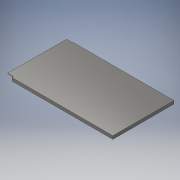
# Autodesk Inventor part: Display Controller
Saved by Autodesk Inventor 2017 SP1 (Build 210196100, 196)
## iProperties
Part Number: Display Controller
Material: Stahl, galvanisiert
Document SubType Name: Modeling
Designer: u26048
Density: 7.85 g/cm^3
Appearance: Galvanisiert
Author: u26048
Autodesk Inventor part; units mm, degrees
ref_plane "YZ Plane" through (0, 0, 0) normal (1, 0, 0) x (0, 1, 0)
ref_plane "XZ Plane" through (0, 0, 0) normal (0, 1, 0) x (-1, 0, 0)
ref_plane "XY Plane" through (0, 0, 0) normal (0, 0, 1) x (1, 0, 0)
sketch "Skizze1" plane through (0, 0, 0) normal (0, 0, 1) x (1, 0, 0)
  line L0 (-83.1, 50.3) -> (83.1, 50.3)
  line L1 (83.1, 50.3) -> (83.1, -50.3)
  line L2 (83.1, -50.3) -> (-83.1, -50.3)
  line L3 (-83.1, -50.3) -> (-83.1, 50.3)
  point P0 (0, 0)
  point P1 (83.1, 0)
  point P2 (0, 50.3)
  dimension "d0" = 166.2
  dimension "d1" = 100.6
  constraints: 8 end point, 2 midpoint, 2 parallel, 1 horizontal, 1 horizontal alignment, 1 perpendicular, 1 vertical alignment
  measures "d0" distance of L1.end L2.end
  measures "d1" distance of L0.end L1.end
extrude "Extrusion1" add sketch "Skizze1" along normal blind 5.26
sketch "Skizze2" plane through (0, 0, 0) normal (0, 0, -1) x (-1, 0, 0)
  line L0 (-83.1, 50.3) -> (-83.1, -50.3) projected
  line L1 (83.1, -50.3) -> (83.1, 50.3) projected
  line L2 (83.1, 50.3) -> (-83.1, 50.3) projected
  line L3 (-70.6, 31.6) -> (-55.6, 31.6)
  line L4 (-55.6, 31.6) -> (-55.6, 39.1)
  line L5 (-55.6, 39.1) -> (-70.6, 39.1)
  line L6 (-70.6, 39.1) -> (-70.6, 31.6)
  line L7 (-70.6, 31.6) -> (-55.6, 39.1) construction
  line L8 (-55.6, 31.6) -> (-70.6, 39.1) construction
  circle A0 centre (-63.1, 35.35) radius 1.5
  line L9 (55.6, 31.6) -> (70.6, 31.6)
  line L10 (70.6, 31.6) -> (70.6, 39.1)
  line L11 (70.6, 39.1) -> (55.6, 39.1)
  line L12 (55.6, 39.1) -> (55.6, 31.6)
  line L13 (55.6, 31.6) -> (70.6, 39.1) construction
  line L14 (70.6, 31.6) -> (55.6, 39.1) construction
  circle A1 centre (63.1, 35.35) radius 1.5
  line L15 (-55.6, -34.05) -> (-55.6, -26.55)
  circle A2 centre (-63.1, -30.3) radius 1.5
  line L16 (-70.6, -34.05) -> (-55.6, -34.05)
  line L17 (-70.6, -34.05) -> (-55.6, -26.55) construction
  line L18 (-55.6, -34.05) -> (-70.6, -26.55) construction
  line L19 (-55.6, -26.55) -> (-70.6, -26.55)
  line L20 (-70.6, -26.55) -> (-70.6, -34.05)
  line L21 (55.6, -26.55) -> (55.6, -34.05)
  circle A3 centre (63.1, -30.3) radius 1.5
  line L22 (70.6, -34.05) -> (70.6, -26.55)
  line L23 (70.6, -26.55) -> (55.6, -26.55)
  line L24 (55.6, -34.05) -> (70.6, -26.55) construction
  line L25 (70.6, -34.05) -> (55.6, -26.55) construction
  line L26 (55.6, -34.05) -> (70.6, -34.05)
  point P0 (0, 0)
  point P1 (63.1, 35.35)
  point P2 (-63.1, -30.3)
  point P3 (63.1, -30.3)
  point P4 (63.1, -30.3)
  dimension "d4" = 20
  dimension "d7" = 126.2
  dimension "d9" = 14.95
  dimension "d10" = 65.65
  dimension "d11" = 15
  dimension "d12" = 7.5
  dimension "d19" = 3
  dimension "d50" = 126.2
  dimension "d57" = 65.65
  constraints: 48 end point, 8 midpoint, 4 centre point, 4 coincident, 2 horizontal, 2 horizontal alignment, 2 parallel, 2 vertical alignment, 1 perpendicular, 1 vertical, 40 other
  measures "d4" distance from line of point (-63.1, 35.35) L0
  measures "d7" distance of point (63.1, 35.35) point (-63.1, 35.35)
  measures "d9" distance from line of L2 point (63.1, 35.35)
  measures "d10" distance of point (63.1, 35.35) point (63.1, -30.3)
  measures "d11" distance of L5.end L4.end
  measures "d12" distance of L4.end L3.end
  measures "d19" diameter of A0
  measures "d50" distance of L3.start L9.start
  measures "d57" distance of L3.end L15.start
extrude "Extrusion2" add sketch "Skizze2" along normal blind 2.5
sketch "Skizze3" plane through (0, 0, 0) normal (0, 0, -1) x (-1, 0, 0)
  line L0 (-82.45, 50.3) -> (82.45, 50.3)
  line L1 (82.45, 50.3) -> (82.45, -50.3)
  line L2 (82.45, -50.3) -> (-82.45, -50.3)
  line L3 (-82.45, -50.3) -> (-82.45, 50.3)
  line L4 (-37.75, 22) -> (-30.25, 22)
  line L5 (-30.25, 22) -> (-30.25, 37)
  line L6 (-30.25, 37) -> (-37.75, 37)
  line L7 (-37.75, 37) -> (-37.75, 22)
  line L8 (-37.75, 22) -> (-30.25, 37) construction
  line L9 (-30.25, 22) -> (-37.75, 37) construction
  circle A0 centre (-34, 29.5) radius 1.25
  line L10 (20.25, 22) -> (27.75, 22)
  line L11 (27.75, 22) -> (27.75, 37)
  line L12 (27.75, 37) -> (20.25, 37)
  line L13 (20.25, 37) -> (20.25, 22)
  line L14 (20.25, 22) -> (27.75, 37) construction
  line L15 (27.75, 22) -> (20.25, 37) construction
  circle A1 centre (24, 29.5) radius 1.25
  line L16 (-37.75, -27) -> (-30.25, -27)
  line L17 (-30.25, -27) -> (-30.25, -12)
  line L18 (-30.25, -12) -> (-37.75, -12)
  line L19 (-37.75, -12) -> (-37.75, -27)
  line L20 (-37.75, -27) -> (-30.25, -12) construction
  line L21 (-30.25, -27) -> (-37.75, -12) construction
  circle A2 centre (-34, -19.5) radius 1.25
  line L22 (20.25, -27) -> (27.75, -27)
  line L23 (27.75, -27) -> (27.75, -12)
  line L24 (27.75, -12) -> (20.25, -12)
  line L25 (20.25, -12) -> (20.25, -27)
  line L26 (20.25, -27) -> (27.75, -12) construction
  line L27 (27.75, -27) -> (20.25, -12) construction
  circle A3 centre (24, -19.5) radius 1.25
  point P0 (0, 0)
  point P1 (-82.45, 0)
  point P2 (0, 50.3)
  point P3 (-34, -19.5)
  point P4 (24, -19.5)
  dimension "d25" = 164.9
  dimension "d26" = 100.6
  dimension "d27" = 48.45
  dimension "d28" = 58
  dimension "d29" = 20.8
  dimension "d30" = 49
  dimension "d31" = 7.5
  dimension "d32" = 15
  dimension "d33" = 2.5
  dimension "d64" = 58
  dimension "d67" = 49
  constraints: 56 end point, 10 midpoint, 4 centre point, 4 coincident, 4 parallel, 3 horizontal, 3 horizontal alignment, 3 vertical alignment, 2 perpendicular, 1 vertical, 39 other
  measures "d25" distance of L1.end L2.end
  measures "d26" distance of L0.end L1.end
  measures "d27" distance from line of point (-34, 29.5) L3
  measures "d28" distance of point (24, 29.5) point (-34, 29.5)
  measures "d29" distance from line of L0 point (24, 29.5)
  measures "d30" distance of point (24, 29.5) point (24, -19.5)
  measures "d31" distance of L6.end L5.end
  measures "d32" distance of L5.end L4.end
  measures "d33" diameter of A0
  measures "d64" distance of L4.start L10.start
  measures "d67" distance of L4.start L16.start
extrude "Extrusion3" add sketch "Skizze3" along normal blind 2.5 contours L7 L6 L5 L4 | L13 L12 L11 L10 | L19 L18 L17 L16 | L25 L24 L23 L22
chamfer "Fase1" distance 2.5 angle 45 16 edges at (70.6, 35.35, -2.5) (55.6, 35.35, -2.5) (34, 22, -2.5) (34, 37, -2.5) (70.6, -30.3, -2.5) (55.6, -30.3, -2.5) (-55.6, -30.3, -2.5) (-70.6, -30.3, -2.5) (-70.6, 35.35, -2.5) (-55.6, 35.35, -2.5) (34, -12, -2.5) (34, -27, -2.5) (-24, -12, -2.5) (-24, -27, -2.5) (-24, 22, -2.5) (-24, 37, -2.5)
sketch "Skizze4" plane through (0, 0, 0) normal (0, 0, -1) x (-1, 0, 0)
  line L0 (-50.25, 45.8) -> (50.25, 45.8) construction
  line L1 (-48.75, 44.3) -> (48.75, 44.3)
  line L2 (48.75, 47.3) -> (-48.75, 47.3)
  arc A0 (-48.75, 47.3) -> (-48.75, 44.3) centre (-48.75, 45.8) ccw
  arc A1 (48.75, 44.3) -> (48.75, 47.3) centre (48.75, 45.8) ccw
  line L3 (-83.1, 50.3) -> (-83.1, -50.3) projected
  line L4 (83.1, 50.3) -> (-83.1, 50.3) projected
  line L5 (-33.1, -43.8) -> (33.1, -43.8) construction
  line L6 (-31.6, -45.3) -> (31.6, -45.3)
  line L7 (31.6, -42.3) -> (-31.6, -42.3)
  arc A2 (-31.6, -42.3) -> (-31.6, -45.3) centre (-31.6, -43.8) ccw
  arc A3 (31.6, -45.3) -> (31.6, -42.3) centre (31.6, -43.8) ccw
  line L8 (-83.1, -50.3) -> (83.1, -50.3) projected
  line L9 (83.1, -50.3) -> (83.1, 50.3) projected
  point P0 (0, 0)
  point P1 (0, 45.8)
  point P2 (0, -43.8)
  dimension "d70" = 100.5
  dimension "d71" = 3
  dimension "d73" = 3
  dimension "d74" = 3
  dimension "d75" = 5
  dimension "d76" = 50
  dimension "d77" = 50
  constraints: 16 end point, 12 point on circle, 8 tangent, 4 centre point, 4 point on line, 2 horizontal, 2 midpoint, 2 parallel, 1 vertical alignment
  measures "d70" distance of L0.start L0.end
  measures "d71" diameter of A1
  measures "d73" distance between parallel lines of L2 L4
  measures "d74" diameter of A3
  measures "d75" distance between parallel lines of L8 L6
  measures "d76" distance from line of L5.start L3
  measures "d77" distance from line of L9 L5.end
extrude "Extrusion4" add sketch "Skizze4" along normal blind 0.5 contours A0 L2 A1 L1 | A2 L7 A3 L6
sketch "Skizze6" plane through (-83.1, -50.3, 0) normal (-1, 0, 0) x (0, 0, 1)
  line L0 (5.26, 100.6) -> (5.26, 0) projected
  line L1 (5.26, 99.6) -> (4.56, 99.6)
  line L2 (4.56, 99.6) -> (4.56, 2.5)
  line L3 (4.56, 2.5) -> (5.26, 2.5)
  line L4 (5.26, 2.5) -> (5.26, 99.6)
  line L5 (0, 0) -> (5.26, 0) projected
  line L6 (0, 100.6) -> (5.26, 100.6) projected
  point P0 (0, 50.3)
  dimension "d83" = 0.7
  dimension "d84" = 2.5
  dimension "d85" = 1
  constraints: 8 end point, 2 parallel, 1 horizontal, 1 perpendicular, 1 point on line
  measures "d83" distance of L3.end L2.end
  measures "d84" distance between parallel lines of L3 L5
  measures "d85" distance between parallel lines of L6 L1
extrude "Extrusion6" add sketch "Skizze6" along normal blind 9.8
equation "\"d77\" = d76"
